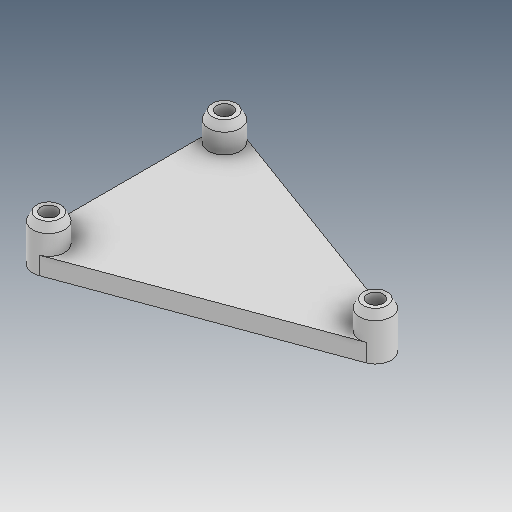
# Autodesk Inventor part: db-25_standoffs_plate
Saved by Autodesk Inventor 2025.1 (Build 291241000, 241)
## iProperties
Created: 2026-06-20
Part Number: db-25_standoffs_plate
Material: Generic
Document SubType Name: Modeling
Designer: Aiden
Density: 1 g/cm^3
Appearance: Default
Author: Aiden
Autodesk Inventor part; units mm, degrees
ref_plane "YZ Plane" through (0, 0, 0) normal (1, 0, 0) x (0, 1, 0)
ref_plane "XZ Plane" through (0, 0, 0) normal (0, 1, 0) x (-1, 0, 0)
ref_plane "XY Plane" through (0, 0, 0) normal (0, 0, 1) x (1, 0, 0)
sketch "Connector Hole Layout" plane through (0, 0, 0) normal (0, 1, 0) x (-1, 0, 0)
  circle A0 centre (42.9488, 7.9638) radius 1.6 construction
  circle A1 centre (-17.5388, 30.2138) radius 1.6 construction
  circle A2 centre (42.9488, 52.4638) radius 1.6 construction
  line L0 (42.9488, 7.9638) -> (42.9488, 52.4638) construction
  line L1 (41.4471, 51.9114) -> (-16.0371, 30.7661) construction
  point P0 (42.9488, 30.2138)
  dimension "d0" = 3.2
  dimension "d22" = 44.5
  dimension "d23" = 61.25
  constraints: 4 end point, 3 coincident, 1 centre point, 1 horizontal alignment, 1 midpoint, 1 vertical, 1 vertical alignment, 10 other
  measures "d0" diameter of A0
  measures "d22" distance of L0.start L0.end
sketch "Sketch8" plane through (0, 0, 0) normal (0, 1, 0) x (-1, 0, 0)
  circle A0 centre (42.9488, 7.9638) radius 1.6 construction
  circle A1 centre (42.9488, 52.4638) radius 1.6 construction
  circle A2 centre (-17.5388, 30.2138) radius 1.6 construction
  circle A3 centre (42.9488, 7.9638) radius 4
  point P0 (0, 0)
  dimension "d51" = 8
  constraints: 4 coincident, 1 centre point
  measures "d51" diameter of A3
extrude "Extrusion5" add sketch "Sketch8" along normal blind 7
sketch "Sketch9" plane through (-42.9488, 7, 7.9638) normal (0, 1, 0) x (1, 0, 0)
  point P0 (42.9488, 7.9638)
  point P1 (0, 0)
hole "Hole2" at (-42.9488, 7, 7.9638) direction (0, -1, 0) diameter 4 depth 5 tip angle 118
chamfer "Chamfer3" distance 1 distance2 2 1 edges at (-38.9488, 7, 7.9638) measured on face at (-39.4488, 7, 7.9638)
pattern_sketch "Sketch Driven Pattern1" from (-42.9488, 0, 7.9638) copies at (-42.9488, 0, 52.4638) at (17.5388, 0, 30.2138)
sketch "Sketch10" plane through (-42.9488, 0, 52.4638) normal (0, -1, 0) x (1, 0, 0)
  circle A0 centre (0, 0) radius 4 projected
  line L0 (1.3809, 3.7541) -> (61.8684, -18.4959)
  circle A1 centre (60.4875, -22.25) radius 4 projected
  line L1 (61.8684, -26.0041) -> (1.3809, -48.2541)
  circle A2 centre (0, -44.5) radius 4 projected
  line L2 (-4, -44.5) -> (-4, 0)
  circle A3 centre (0, 0) radius 4 projected
  circle A4 centre (0, -44.5) radius 4 projected
  point P0 (42.9488, -52.4638)
  constraints: 6 end point, 6 point on circle, 5 tangent, 2 other
extrude "Extrusion6" add sketch "Sketch10" along normal blind 4.5
body "Solid2"
